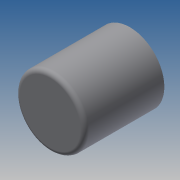
# Autodesk Inventor part: Knopp
Saved by Autodesk Inventor 2019 (Build 230136000, 136)
## iProperties
Created: 2022-10-31
Part Number: Knopp
Material: Generisch
Document SubType Name: Modeling
Designer: Dominik Schmidt
Density: 1 g/cm^3
Appearance: Vorgabe
Author: Dominik Schmidt
Autodesk Inventor part; units mm, degrees
ref_plane "YZ Plane" through (0, 0, 0) normal (1, 0, 0) x (0, 1, 0)
ref_plane "XZ Plane" through (0, 0, 0) normal (0, 1, 0) x (-1, 0, 0)
ref_plane "XY Plane" through (0, 0, 0) normal (0, 0, 1) x (1, 0, 0)
sketch "Skizze1" plane through (0, 0, 0) normal (0, 0, 1) x (1, 0, 0)
  circle A0 centre (0, 0) radius 8.5 projected
  circle A1 centre (0, 0) radius 3.7 projected
  circle A2 centre (0, 0) radius 8
  circle A3 centre (0, 0) radius 5.85
  point P0 (0, 0)
  dimension "d0" = 16
  dimension "d1" = 11.7
  constraints: 2 centre point, 2 coincident
  measures "d0" diameter of A2
  measures "d1" diameter of A3
extrude "Extrusion1" add sketch "Skizze1" along normal blind 3 contours A2
sketch "Skizze2" plane through (0, 0, 3) normal (0, 0, 1) x (1, 0, 0)
  circle A0 centre (0, 0) radius 3.05
  circle A1 centre (0, 0) radius 8.1333
  dimension "d4" = 6.1
  constraints: 2 centre point, 2 coincident
  measures "d4" diameter of A0
extrude "Extrusion2" add sketch "Skizze2" along normal blind 15
sketch "Skizze3" plane through (0, 0, 18) normal (0, 0, 1) x (1, 0, 0)
  circle A0 centre (0, 0) radius 8.1333 projected
extrude "Extrusion3" add sketch "Skizze3" along normal blind 0.5
fillet "Rundung1" radius 1 1 edges at (-8.1333, 0, 18.5)
